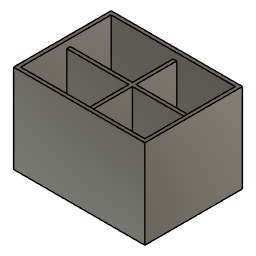
10408김준호_보관함 (Autodesk Fusion 360 design; units mm, degrees)
Autodesk Fusion 360 part; units mm, degrees
box "상자 기본체2" add length 55 width 74 height 50 placed x (0, 1, 0) y (-1, 0, 0) z (0, 0, 1) at (49, -25, 0)
shell "쉘1" thickness 2 removed faces 1 at (-0.3333, -6.6667, 50)
box "상자 기본체3" add length 2 width 70 height 1 placed x (0, -1, 0) y (1, 0, 0) z (0, 0, 1) at (-23, 5, 2)
box "상자 기본체4" cut length 51 width 2 height 1 placed x (0, -1, 0) y (1, 0, 0) z (0, 0, 1) at (12, 28, 2)
box "상자 기본체5" add length 51 width 2 height 1 placed x (0, 1, 0) y (-1, 0, 0) z (0, 0, 1) at (14, -23, 2)
extrude "돌출1" add 1 faces at (0.3333, 3.6667, 3) along direction (0, 0, 1) blind 43
